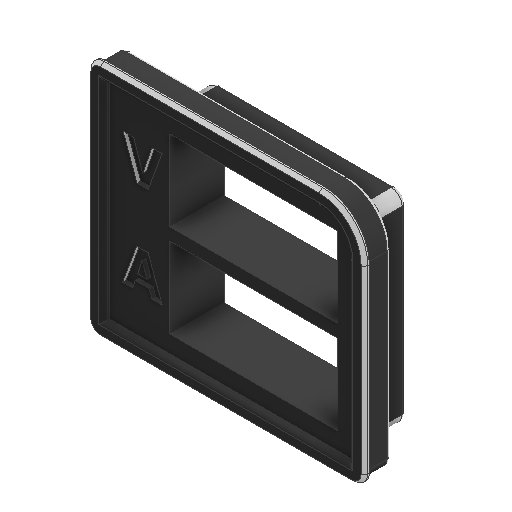
# Autodesk Inventor part: display_cover_2mm
Saved by Autodesk Inventor 2025 (Build 290162000, 162)
## iProperties
Created: 2025-01-08
Part Number: display_cover_2mm
Material: Generic
Document SubType Name: Modeling
Designer: Jan Mareš
Density: 1 g/cm^3
Appearance: Default
Author: Jan Mareš
Autodesk Inventor part; units mm, degrees
ref_plane "YZ Plane" through (0, 0, 0) normal (1, 0, 0) x (0, 1, 0)
ref_plane "XZ Plane" through (0, 0, 0) normal (0, 1, 0) x (-1, 0, 0)
ref_plane "XY Plane" through (0, 0, 0) normal (0, 0, 1) x (1, 0, 0)
sketch "Sketch1" plane through (0, 0, 0) normal (0, 0, 1) x (1, 0, 0)
  line L0 (0, -35) -> (0, 35) construction
  line L1 (-42, 0) -> (42, 0) construction
  line L2 (-30, 25) -> (30, 25)
  line L3 (30, 25) -> (30, -25)
  line L4 (30, -25) -> (-30, -25)
  line L5 (-30, -25) -> (-30, 25)
  line L6 (-30, 0) -> (30, 0) construction
  point P0 (0, 0)
  dimension "d0" = 60
  dimension "d1" = 50
  constraints: 10 end point, 3 midpoint, 2 parallel, 1 horizontal, 1 perpendicular
  measures "d0" distance of L2.start L2.end
  measures "d1" distance of L2.end L3.end
extrude "Extrusion1" add sketch "Sketch1" along normal blind 7
sketch "Sketch2" plane through (0, 0, 7) normal (0, 0, 1) x (1, 0, 0)
  line L0 (-25, 19.4999) -> (-25, -19.4974) construction
  arc A0 (-23, 21.4999) -> (-25, 19.4999) centre (-23, 19.4999) ccw construction
  arc A1 (-25, -19.4974) -> (-23, -21.4974) centre (-23, -19.4974) ccw construction
  line L1 (-23, -21.4974) -> (22.9999, -21.4973) construction
  arc A2 (22.9999, -21.4973) -> (24.9999, -19.4974) centre (22.9999, -19.4974) ccw construction
  arc A3 (21, 13.4999) -> (16.9999, 17.5) centre (16.9999, 13.4999) ccw projected
  line L2 (-16.9999, 17.5) -> (16.9999, 17.5) projected
  line L3 (21, 13.4999) -> (21, -13.4973) projected
  arc A4 (16.9999, -17.4974) -> (21, -13.4973) centre (16.9999, -13.4973) ccw projected
  line L4 (16.9999, -17.4974) -> (-16.9999, -17.4974) projected
  arc A5 (-21, -13.4973) -> (-16.9999, -17.4974) centre (-16.9999, -13.4973) ccw projected
  line L5 (-21, -13.4973) -> (-21, 13.4999) projected
  arc A6 (-16.9999, 17.5) -> (-21, 13.4999) centre (-16.9999, 13.4999) ccw projected
  line L6 (24.9999, 13.4999) -> (24.9999, -50.4974) construction
  arc A7 (24.9999, 13.4999) -> (16.9999, 21.4999) centre (16.9999, 13.4999) ccw construction
  line L7 (16.9999, 21.4999) -> (-23, 21.4999) construction
  line L8 (24.7499, -19.4974) -> (24.7499, 13.4999)
  arc A8 (24.7499, 13.4999) -> (16.9999, 21.2499) centre (16.9999, 13.4999) ccw
  line L9 (16.9999, 21.2499) -> (-23, 21.2499)
  arc A9 (-23, 21.2499) -> (-24.75, 19.4999) centre (-23, 19.4999) ccw
  line L10 (-24.75, 19.4999) -> (-24.75, -19.4974)
  arc A10 (-24.75, -19.4974) -> (-23, -21.2473) centre (-23, -19.4974) ccw
  line L11 (-23, -21.2473) -> (22.9999, -21.2473)
  arc A11 (22.9999, -21.2473) -> (24.7499, -19.4974) centre (22.9999, -19.4974) ccw
  line L12 (24.4141, -20.9116) -> (24.2374, -20.7348) construction
  arc A12 (39.7499, 13.4999) -> (16.9999, 36.2499) centre (16.9999, 13.4999) ccw
  line L13 (39.7499, 13.4999) -> (39.7499, -19.4974)
  arc A13 (22.9999, -36.2473) -> (39.7499, -19.4974) centre (22.9999, -19.4974) ccw
  line L14 (22.9999, -36.2473) -> (-23, -36.2473)
  arc A14 (-39.75, -19.4974) -> (-23, -36.2473) centre (-23, -19.4974) ccw
  line L15 (-39.75, -19.4974) -> (-39.75, 19.4999)
  arc A15 (-23, 36.2499) -> (-39.75, 19.4999) centre (-23, 19.4999) ccw
  line L16 (-23, 36.2499) -> (16.9999, 36.2499)
  point P0 (0, 0)
  dimension "d27" = 0.25
  dimension "d29" = 15
  constraints: 18 end point, 18 point on circle, 8 centre point, 1 line through centre, 13 other
  measures "d27" distance between parallel lines of L6 L8
  measures "d29" distance between parallel lines of L9 L16
extrude "Extrusion2" cut sketch "Sketch2" against normal up to next contours L13 A13 L14 A14 L15 A15 L16 A12
sketch "Sketch3" plane through (0, 0, 7) normal (0, 0, 1) x (1, 0, 0)
  arc A0 (16.9999, -17.4973) -> (21, -13.4973) centre (16.9999, -13.4973) ccw construction
  line L0 (21, 13.4999) -> (21, -13.4973) construction
  arc A1 (21, 13.4999) -> (16.9999, 17.5) centre (16.9999, 13.4999) ccw construction
  line L1 (-16.9999, 17.5) -> (16.9999, 17.5) construction
  arc A2 (-16.9999, 17.5) -> (-21, 13.4999) centre (-16.9999, 13.4999) ccw construction
  line L2 (-21, -13.4973) -> (-21, 13.4999) construction
  arc A3 (-21, -13.4973) -> (-16.9999, -17.4973) centre (-16.9999, -13.4973) ccw construction
  line L3 (16.9999, -17.4973) -> (-16.9999, -17.4973) construction
  line L4 (-22.5, -19) -> (22.5, -19) projected
  line L5 (-22.5, 19) -> (-22.5, -19) projected
  line L6 (16.9999, 19) -> (-22.5, 19) projected
  arc A4 (22.5, 13.4999) -> (16.9999, 19) centre (16.9999, 13.4999) ccw projected
  line L7 (22.5, -19) -> (22.5, 13.4999) projected
  point P0 (0, 0)
extrude "Extrusion3" cut sketch "Sketch3" against normal blind 1.1
sketch "Sketch4" plane through (0, 0, 0) normal (0, 0, -1) x (-1, 0, 0)
  line L0 (-19, 15.5026) -> (11, 15.5026) construction
  line L1 (11, 1.5026) -> (-19, 1.5026) construction
  line L2 (-19, 1.5026) -> (-19, 15.5026) construction
  line L3 (11, 15.5026) -> (11, 1.5026) construction
  line L4 (11, -1.4974) -> (11, -15.4974) construction
  line L5 (-19, -1.4974) -> (11, -1.4974) construction
  line L6 (11, -15.4974) -> (-19, -15.4974) construction
  line L7 (-19, -15.4974) -> (-19, -1.4974) construction
  line L8 (14, 18.5026) -> (-22, 18.5026)
  line L9 (-22, 18.5026) -> (-22, -18.4974)
  line L10 (-22, -18.4974) -> (14, -18.4974)
  line L11 (14, -18.4974) -> (14, 18.5026)
  line L12 (-4, -18.4974) -> (-4, -15.4974) construction
  line L13 (-4, 18.5026) -> (-4, 15.5026) construction
  line L14 (-19, 8.5026) -> (-22, 8.5026) construction
  line L15 (11, 8.5026) -> (14, 8.5026) construction
  point P0 (0, 0)
  dimension "d10" = 3
  constraints: 16 end point, 6 midpoint, 4 perpendicular, 3 point on line, 2 parallel, 1 horizontal, 1 vertical
  measures "d10" distance of L14.start L14.end
extrude "Extrusion4" add sketch "Sketch4" along normal blind 4
sketch "Sketch5" plane through (0, 0, 5.9) normal (0, 0, 1) x (1, 0, 0)
  line L0 (-11, -15.4974) -> (19, -15.4974) construction
  line L1 (-11, -1.4974) -> (-11, -15.4974) construction
  line L2 (19, -15.4974) -> (19, -1.4974) construction
  line L3 (19, -1.4974) -> (-11, -1.4974) construction
  line L4 (19, 1.5026) -> (19, 15.5026) construction
  line L5 (-11, 1.5026) -> (19, 1.5026) construction
  line L6 (-11, 15.5026) -> (-11, 1.5026) construction
  line L7 (19, 15.5026) -> (-11, 15.5026) construction
  line L8 (19.35, -15.8474) -> (-11.35, -15.8474)
  line L9 (-11.35, -15.8474) -> (-11.35, -1.1474)
  line L10 (-11.35, -1.1474) -> (19.35, -1.1474)
  line L11 (19.35, -1.1474) -> (19.35, -15.8474)
  line L12 (19.35, 1.1526) -> (19.35, 15.8526)
  line L13 (19.35, 15.8526) -> (-11.35, 15.8526)
  line L14 (-11.35, 15.8526) -> (-11.35, 1.1526)
  line L15 (-11.35, 1.1526) -> (19.35, 1.1526)
  point P0 (0, 0)
  dimension "d13" = 0.35
  dimension "d14" = 0.35
  constraints: 16 end point, 6 other
  measures "d13" distance between parallel lines of L0 L8
  measures "d14" distance between parallel lines of L5 L15
extrude "Extrusion5" cut sketch "Sketch5" against normal up to next
sketch "Sketch13" plane through (0, 0, 0) normal (0, 0, -1) x (-1, 0, 0)
  line L0 (25.27, -11.6524) -> (25.91, -11.6524) construction
  line L1 (25.91, -12.2924) -> (25.91, -11.6524) construction
  line L2 (25.27, -12.2924) -> (25.91, -12.2924) construction
  line L3 (25.27, -11.6524) -> (25.27, -12.2924) construction
  line L4 (23.37, -11.6524) -> (23.37, -12.2924) construction
  line L5 (22.73, -12.2924) -> (23.37, -12.2924) construction
  line L6 (22.73, -11.6524) -> (22.73, -12.2924) construction
  line L7 (23.37, -11.6524) -> (22.73, -11.6524) construction
  line L8 (20.19, -12.2924) -> (20.83, -12.2924) construction
  line L9 (20.83, -11.6524) -> (20.83, -12.2924) construction
  line L10 (20.83, -11.6524) -> (20.19, -11.6524) construction
  line L11 (20.19, -11.6524) -> (20.19, -12.2924) construction
  line L12 (18.29, -11.6524) -> (18.29, -12.2924) construction
  line L13 (17.65, -12.2924) -> (18.29, -12.2924) construction
  line L14 (17.65, -11.6524) -> (17.65, -12.2924) construction
  line L15 (18.29, -11.6524) -> (17.65, -11.6524) construction
  line L16 (14, -18.4974) -> (14, 18.5026) projected
  line L17 (14, 18.5026) -> (14, -18.4974) projected
  line L18 (-22, -18.4974) -> (14, -18.4974) projected
  line L19 (-22, 18.5026) -> (-22, -18.4974) projected
  line L20 (-22, 18.5026) -> (14, 18.5026) projected
  line L21 (30, -26.4974) -> (-30, -26.4974)
  line L22 (-30, -26.4974) -> (-30, 26.5026)
  line L23 (-30, 26.5026) -> (30, 26.5026)
  line L24 (30, 26.5026) -> (30, -26.4974)
  point P0 (0, 0)
  dimension "d52" = 8
  dimension "d53" = 16
  dimension "d54" = 8
  dimension "d55" = 8
  constraints: 8 end point, 2 parallel, 1 horizontal, 1 perpendicular
  measures "d52" distance between parallel lines of L21 L18
  measures "d53" distance between parallel lines of L16 L24
  measures "d54" distance between parallel lines of L19 L22
  measures "d55" distance between parallel lines of L23 L20
extrude "Extrusion6" cut sketch "Sketch13" against normal blind 1.5
sketch "Sketch12" plane through (0, 0, 5.9) normal (0, 0, 1) x (1, 0, 0)
  line L0 (-21, -13.4973) -> (-21, 13.4999) construction
  line L1 (-11.35, 1.1526) -> (-11.35, 15.8526) construction
  line L2 (-11.35, -15.8474) -> (-11.35, -1.1474) construction
  line L3 (-20.1443, -4.9695) -> (-12.75, -4.9695) construction
  line L4 (-12.75, -4.9695) -> (-12.75, -11.9503) construction
  line L5 (-12.75, -11.9503) -> (-20.1443, -11.9503) construction
  line L6 (-20.1443, -11.9503) -> (-20.1443, -4.9695) construction
  line L7 (-11.35, 8.5026) -> (-21, 8.5026) construction
  line L8 (-21, -2.6195) -> (-11.35, -2.6195) construction
  line L9 (-11.35, -8.4974) -> (-21, -8.4974) construction
  line L10 (-11.35, -11.9974) -> (-21, -11.9974) construction
  line L11 (-21, 5.0026) -> (-11.35, 5.0026) construction
  line L12 (-16.175, 8.5026) -> (-16.175, -15.0992) construction
  line L13 (-22.5, -19) -> (-22.5, 19) projected
  line L14 (-20.05, 12.0287) -> (-12.75, 12.0287) construction
  line L15 (-12.75, 12.0287) -> (-12.75, 5.0026) construction
  line L16 (-12.75, 5.0026) -> (-20.05, 5.0026) construction
  line L17 (-20.05, 5.0026) -> (-20.05, 12.0287) construction
  line L18 (-12.7843, -11.9695) -> (-14.6471, -11.9695)
  line L19 (-14.6471, -11.9695) -> (-15.1329, -10.5581)
  line L20 (-15.1329, -10.5581) -> (-17.7214, -10.5581)
  line L21 (-17.7214, -10.5581) -> (-18.2071, -11.9695)
  line L22 (-18.2071, -11.9695) -> (-20.03, -11.9695)
  line L23 (-20.03, -11.9695) -> (-17.4471, -4.9695)
  line L24 (-17.4471, -4.9695) -> (-15.3671, -4.9695)
  line L25 (-15.3671, -4.9695) -> (-12.7843, -11.9695)
  line L26 (-15.5671, -9.2724) -> (-16.43, -6.7695)
  line L27 (-16.43, -6.7695) -> (-17.2871, -9.2724)
  line L28 (-17.2871, -9.2724) -> (-15.5671, -9.2724)
  line L29 (-12.81, 12.0287) -> (-15.3643, 5.0287)
  line L30 (-15.3643, 5.0287) -> (-17.3814, 5.0287)
  line L31 (-17.3814, 5.0287) -> (-19.9357, 12.0287)
  line L32 (-19.9357, 12.0287) -> (-18.0443, 12.0287)
  line L33 (-18.0443, 12.0287) -> (-16.3529, 7.1145)
  line L34 (-16.3529, 7.1145) -> (-14.6614, 12.0287)
  line L35 (-14.6614, 12.0287) -> (-12.81, 12.0287)
  point P0 (0, 0)
  point P1 (-19.8647, 12.0013)
  dimension "d46" = 3.5
  dimension "d62" = 7.3943
  dimension "d64" = 1.4
  dimension "d65" = 7.3
  dimension "d66" = 3.5
  dimension "d67" = 7.0261
  dimension "d68" = 1.4
  constraints: 12 end point, 6 point on line, 4 perpendicular, 3 midpoint, 1 horizontal, 1 parallel, 4 other
  measures "d46" distance between parallel lines of L9 L10
  measures "d62" distance of L3.start L3.end
  measures "d64" distance between parallel lines of L2 L4
  measures "d65" distance of L17.end L14.end
  measures "d66" distance between parallel lines of L16 L7
  measures "d67" distance of L17.start L17.end
  measures "d68" distance between parallel lines of L1 L15
emboss "Emboss1" sketch "Sketch12" operation cut depth 0.7 direction (0, 0, -1)
fillet "Fillet3" radius 2 4 edges at (-14, -18.4974, -1.25) (-14, 18.5026, -1.25) (22, 18.5026, -1.25) (22, -18.4974, -1.25)
fillet "Fillet2" radius 0.75 29 edges at (4, -18.4974, -4) (-14, 0.0026, -4) (4, 18.5026, -4) (22, 0.0026, -4) (-22.5, 0, 7) (0, -19, 7) (20.8891, 17.3891, 7) (-2.75, 19, 7) (22.5, -2.75, 7) (-24.2374, -20.7348, 1.5) (0, -21.2473, 1.5) (24.2374, -20.7348, 1.5) (24.7499, -2.9987, 1.5) (22.48, 18.98, 1.5) (-3, 21.2499, 1.5) (-24.2374, 20.7374, 1.5) (-24.75, 0.0013, 1.5) (-13.4142, 17.9169, 1.5) (4, 18.5026, 1.5) (21.4142, 17.9169, 1.5) (22, 0.0026, 1.5) (21.4142, -17.9116, 1.5) (4, -18.4974, 1.5) (-13.4142, -17.9116, 1.5) (-14, 0.0026, 1.5) (-13.4142, 17.9169, -4) (-13.4142, -17.9116, -4) (21.4142, -17.9116, -4) (21.4142, 17.9169, -4)
sketch "Sketch11" plane through (0, 0, 0) normal (0, 1, 0) x (-1, 0, 0)
  line L0 (24.75, 7) -> (23, 7) construction
  line L1 (24.75, 7) -> (24.75, 0) construction
  line L2 (23, 7.1) -> (25, 7.1) construction
  line L3 (24.75, 7) -> (25.3, 6.3445)
  line L4 (25.3, 6.3445) -> (25.3, 6.0445)
  line L5 (24.75, 7) -> (24.75, 5.583)
  line L6 (25.3, 6.0445) -> (24.75, 5.583)
  point P0 (0, 0)
  dimension "d38" = 50
  dimension "d39" = 40
  dimension "d40" = 0.3
  constraints: 8 end point, 1 point on line, 1 vertical
  measures "d38" angle of L1 L6
  measures "d39" angle of L1 L3
  measures "d40" distance of L3.end L4.end
sketch3d "3D Sketch3"
  line L0 (-24.75, -19.4974, 7) -> (-24.75, 19.4999, 7)
  arc A0 (-24.75, 19.4999, 7) -> (-23, 21.2499, 7) centre (-23, 19.4999, 7) ccw
  line L1 (-23, 21.2499, 7) -> (16.9999, 21.2499, 7)
  arc A1 (16.9999, 21.2499, 7) -> (24.7499, 13.4999, 7) centre (16.9999, 13.4999, 7) ccw
  line L2 (24.7499, 13.4999, 7) -> (24.7499, -19.4974, 7)
  arc A2 (24.7499, -19.4974, 7) -> (22.9999, -21.2473, 7) centre (22.9999, -19.4974, 7) ccw
  line L3 (22.9999, -21.2473, 7) -> (-23, -21.2473, 7)
  arc A3 (-23, -21.2473, 7) -> (-24.75, -19.4974, 7) centre (-23, -19.4974, 7) ccw
sweep "Sweep3" add profiles "Sketch11" path "3D Sketch3"
body "Solid1"
